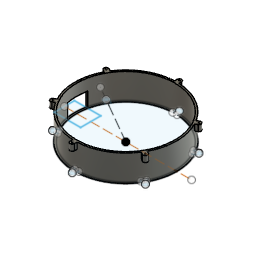
volute v1 (Autodesk Fusion 360 design; units mm, degrees)
Autodesk Fusion 360 part; units mm, degrees
sketch "Sketch1" plane through (0, 0, 0) normal (0, 1, 0) x (1, 0, 0)
  circle A0 centre (0, 0) radius 56
  circle A1 centre (0, 0) radius 58
  line L0 (-70, 0) -> (75, 0) construction
  line L1 (-70, 11.5) -> (-40, 11.5)
  line L2 (-40, 11.5) -> (-40, -11.5)
  line L3 (-40, -11.5) -> (-70, -11.5)
  line L4 (-70, -11.5) -> (-70, 11.5)
  line L5 (0, 0) -> (-68.4625, 39.5268) construction
  line L6 (-47.1991, 30.1371) -> (-51.611, 32.6844)
  arc A2 (-51.611, 32.6844) -> (-54.111, 28.3542) centre (-52.861, 30.5193) ccw
  line L7 (-54.111, 28.3542) -> (-49.6991, 25.807)
  line L8 (-45.8504, 26.4717) -> (-52.861, 30.5193) construction
  circle A3 centre (-52.861, 30.5193) radius 1
  line L9 (-49.6991, -25.807) -> (-54.111, -28.3542)
  circle A4 centre (-52.861, -30.5193) radius 1
  line L10 (-51.611, -32.6844) -> (-47.1991, -30.1371)
  arc A5 (-54.111, -28.3542) -> (-51.611, -32.6844) centre (-52.861, -30.5193) ccw
  line L11 (-2.5, -55.9442) -> (-2.5, -61.0386)
  circle A6 centre (0, -61.0386) radius 1
  line L12 (2.5, -61.0386) -> (2.5, -55.9442)
  arc A7 (-2.5, -61.0386) -> (2.5, -61.0386) centre (0, -61.0386) ccw
  line L13 (47.1991, -30.1371) -> (51.611, -32.6844)
  circle A8 centre (52.861, -30.5193) radius 1
  line L14 (54.111, -28.3542) -> (49.6991, -25.807)
  arc A9 (51.611, -32.6844) -> (54.111, -28.3542) centre (52.861, -30.5193) ccw
  line L15 (49.6991, 25.807) -> (54.111, 28.3542)
  circle A10 centre (52.861, 30.5193) radius 1
  line L16 (51.611, 32.6844) -> (47.1991, 30.1371)
  arc A11 (54.111, 28.3542) -> (51.611, 32.6844) centre (52.861, 30.5193) ccw
  line L17 (2.5, 55.9442) -> (2.5, 61.0386)
  circle A12 centre (0, 61.0386) radius 1
  line L18 (-2.5, 61.0386) -> (-2.5, 55.9442)
  arc A13 (2.5, 61.0386) -> (-2.5, 61.0386) centre (0, 61.0386) ccw
  circle A14 centre (-52.861, -30.5193) radius 0.75
  circle A15 centre (0, -61.0386) radius 0.75
  circle A16 centre (52.861, -30.5193) radius 0.75
  circle A17 centre (52.861, 30.5193) radius 0.75
  circle A18 centre (0, 61.0386) radius 0.75
  circle A19 centre (-52.861, 30.5193) radius 0.75
  dimension "d30" = 112
  dimension "d31" = 116
  dimension "d32" = 23
  dimension "d33" = 5
  dimension "d34" = 30
  dimension "d35" = 2
  dimension "d37" = 360
  dimension "d42" = 1.5
  dimension "d44" = 360
  constraint coincident A0.centre A1.centre
  constraint horizontal L0
  constraint parallel L0 L1
  constraint perpendicular L1 L2
  constraint perpendicular L2 L3
  constraint perpendicular L1 L4
  constraint symmetric L0 L1 L3
  constraint tangent L6 A2
  constraint tangent A2 L7
  constraint parallel L6 L7
  constraint coincident L5 A2.centre
  constraint parallel L5 L8
  constraint coincident L5 L8.start
  constraint coincident A0 L6.start
  constraint coincident A0 L7.end
  constraint concentric A2 A3
  constraint concentric A4 A14
  measures "d30" diameter of A0
  measures "d31" diameter of A1
  measures "d32" distance of L1 L3
  measures "d33" diameter of A2
  measures "d34" angle of L0 L5
  measures "d35" diameter of A3
  measures "d42" diameter of A14
extrude "Extrude1" add sketch "Sketch1" along normal blind 30 contours A0 A1 L14 L15 | A0 A1 L15 L16 | A0 A1 L13 L14 | A0 A1 L16 L17 | A0 A1 L12 L13 | A0 A1 L17 L18 | A0 A1 L11 L12 | A0 A1 L6 L18 | A0 A1 L10 L11 | A0 A1 L6 L7 | A0 A1 L9 L10 | A0 A1 L1 L7 | A0 A1 L3 L9 | A0 A1 L1 L3
extrude "Extrude2" add sketch "Sketch1" along normal blind 2 contours A0 A1 L15 L16 | A0 A1 L13 L14 | A1 L15 L16 A11 | A1 L13 L14 A9 | A0 A1 L17 L18 | A0 A1 L11 L12 | A1 L17 L18 A13 | A1 L11 L12 A7 | A0 A1 L6 L7 | A0 A1 L9 L10 | A1 L6 A2 L7 | A1 L9 L10 A5
extrude "Extrude3" add sketch "Sketch1" against normal blind 7 from surface at 30 contours A1 L15 L16 A11 | A1 L13 L14 A9 | A1 L17 L18 A13 | A1 L11 L12 A7 | A1 L6 A2 L7 | A1 L9 L10 A5 | A3 | A4 | A6 | A8 | A10 | A12
extrude "Extrude4" cut sketch "Sketch1" along normal blind 17 contours A0 A1 L1 L3
fillet "Fillet1" radius 1 2 edges at (-2.5, 1, 57.9461) (2.5, 1, 57.9461)
fillet "Fillet1" radius 1 1 edges at (0, 2, 58)
fillet "Fillet2" radius 1 3 edges at (48.9328, 1, 31.1381) (50.2295, 2, 29) (51.4328, 1, 26.808)
fillet "Fillet3" radius 1 12 edges at (48.9328, 1, -31.1381) (50.2295, 2, -29) (51.4328, 1, -26.808) (-2.5, 1, -57.9461) (0, 2, -58) (2.5, 1, -57.9461) (-51.4328, 1, -26.808) (-50.2295, 2, -29) (-48.9328, 1, -31.1381) (-50.2295, 2, 29) (-48.9328, 1, 31.1381) (-51.4328, 1, 26.808)
named bodies: "volute"
